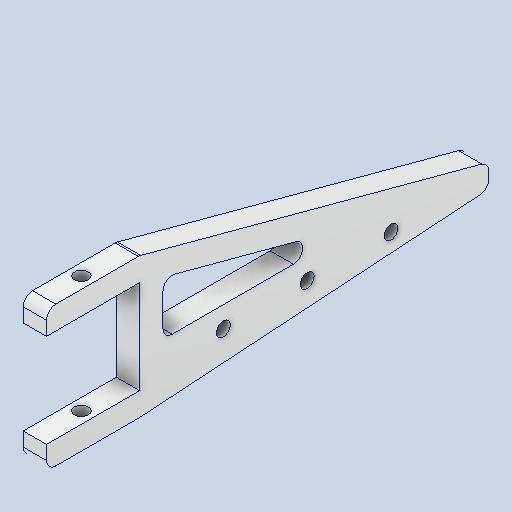
# Autodesk Inventor part: base_weel-v2-Plate-7
Saved by Autodesk Inventor 2025.2 (Build 292293000, 293)
## iProperties
Created: 2025-01-14
Part Number: base_weel-v2-Plate-7
Material: アルミニウム 6061
Document SubType Name: Modeling
Designer: haruy
Density: 2.7 g/cm^3
Appearance: アルミニウム - フラット
Author: haruy
Autodesk Inventor part; units mm, degrees
ref_plane "YZ Plane" through (0, 0, 0) normal (1, 0, 0) x (0, 1, 0)
ref_plane "XZ Plane" through (0, 0, 0) normal (0, 1, 0) x (-1, 0, 0)
ref_plane "XY Plane" through (0, 0, 0) normal (0, 0, 1) x (1, 0, 0)
sketch "スケッチ1" plane through (0, 0, 0) normal (1, 0, 0) x (0, 1, 0)
  line L0 (0, 0) -> (20.1, 0)
  line L1 (20.1, 0) -> (20.1, -20)
  line L2 (20.1, -20) -> (0, -20)
  line L3 (0, -20) -> (0, 0)
  line L4 (0, -20) -> (5, -20)
  line L5 (5, -20) -> (5, -95)
  line L6 (5, -95) -> (0, -95)
  line L7 (0, -95) -> (0, -20)
  circle A0 centre (2.5, -38) radius 1.5
  circle A1 centre (2.5, -56) radius 1.5
  circle A2 centre (2.5, -74) radius 1.5
  line L8 (20.1, 0) -> (25.1, 0)
  line L9 (25.1, 0) -> (25.1, -20)
  line L10 (25.1, -20) -> (20.1, -20)
  line L11 (20.1, -20) -> (20.1, 0)
  line L12 (0, 0) -> (-5, 0)
  line L13 (-5, 0) -> (-5, -20)
  line L14 (-5, -20) -> (0, -20)
  line L15 (0, -20) -> (0, 0)
  line L16 (25.1, -20) -> (5, -95)
  line L17 (-5, -20) -> (0, -95)
  line L18 (25.1, -25) -> (15.1, -25)
  line L19 (15.1, -25) -> (15.1, 0.1)
  line L20 (0, -25) -> (25.1, -25)
  line L21 (25.1, -25) -> (25.1, 0.1)
  line L22 (20.2704, -18.7057) -> (0.1704, -93.7057)
  line L23 (7, -95) -> (7, -18)
  line L24 (7, -18) -> (0, -18)
  line L25 (0, -35) -> (-35, -35)
  line L26 (-35, -35) -> (-35, -85)
  line L27 (-35, -85) -> (0, -85)
  line L28 (0, -85) -> (0, -35)
  line L29 (-35, -38) -> (-70, -38)
  line L30 (-70, -38) -> (-70, -82)
  line L31 (-70, -82) -> (-35, -82)
  line L32 (-35, -82) -> (-35, -38)
  line L33 (7.5, -95) -> (-2.5, -95)
  line L34 (-2.5, -95) -> (-2.5, -21)
  line L35 (-2.5, -21) -> (7.5, -21)
  line L36 (7.5, -21) -> (7.5, -95)
  line L37 (-2.5, -21) -> (-64, -21)
  line L38 (-64, -21) -> (-64, -31)
  line L39 (-64, -31) -> (-2.5, -31)
  line L40 (-2.5, -31) -> (-2.5, -21)
  point P0 (7, -25)
  point P1 (18.5836, -25)
  point P2 (7, -68.2222)
  dimension "d0" = 20.1
  dimension "d1" = 20
  dimension "d2" = 5
  dimension "d3" = 75
  dimension "d4" = 3
  dimension "d5" = 3
  dimension "d6" = 3
  dimension "d7" = 2.5
  dimension "d8" = 2.5
  dimension "d9" = 2.5
  dimension "d10" = 18
  dimension "d11" = 18
  dimension "d12" = 18
  dimension "d13" = 5
  dimension "d14" = 5
  dimension "d15" = 0
  dimension "d16" = 0
  dimension "d17" = 5
  dimension "d18" = 5
  dimension "d19" = 5
  dimension "d20" = 2
  dimension "d33" = 50
  dimension "d34" = 35
  dimension "d35" = 35
  dimension "d36" = 44
  dimension "d37" = 3
  dimension "d38" = 0
  dimension "d39" = 10
  dimension "d40" = 0
  dimension "d41" = 5
  dimension "d42" = 5
  dimension "d43" = 6
  dimension "d44" = 10
  dimension "d46" = 1
  constraints: 82 end point, 17 parallel, 9 perpendicular, 8 horizontal, 3 centre point, 1 point on line, 3 other
  measures "d0" distance of L1.end L2.end
  measures "d1" distance of L0.end L1.end
  measures "d2" distance of L5.end L6.end
  measures "d3" distance between parallel lines of L6 L2
  measures "d4" diameter of A0
  measures "d5" diameter of A1
  measures "d6" diameter of A2
  measures "d7" distance from line of A0.centre L7
  measures "d8" distance from line of A1.centre L7
  measures "d9" distance from line of A2.centre L7
  measures "d10" distance from line of A0.centre L2
  measures "d11" distance of A1.centre A0.centre
  measures "d12" distance of A2.centre A1.centre
  measures "d13" distance of L9.end L10.end
  measures "d14" distance of L14.end L13.end
  measures "d15" distance between parallel lines of L10 L2
  measures "d16" distance between parallel lines of L4 L14
  measures "d17" distance between parallel lines of L10 L18
  measures "d18" distance between parallel lines of L2 L20
  measures "d19" distance between parallel lines of L16 L22
  measures "d20" distance between parallel lines of L5 L23
  measures "d33" distance of L26.end L25.end
  measures "d34" distance of L25.start L25.end
  measures "d35" distance of L31.end L30.end
  measures "d36" distance of L30.end L29.end
  measures "d37" distance between parallel lines of L25 L29
  measures "d38" distance between parallel lines of L7 L28
  measures "d39" distance between parallel lines of L6 L27
  measures "d40" distance between parallel lines of L6 L33
  measures "d41" distance from line of L36 A2.centre
  measures "d42" distance from line of L34 A2.centre
  measures "d43" distance between parallel lines of L30 L38
  measures "d44" distance between parallel lines of L39 L37
  measures "d46" distance between parallel lines of L35 L4
extrude "押し出し1" add sketch "スケッチ1" against normal blind 5 contours L3 L14 L13 L12 | L8 L9 L10 L1 | L19 L20 L36 L35 L23 L2 | L2 L22 L18 L19 | L2 L5 L35 L7 | L7 L35 L37 L17 L14 | L2 L10 L16 L18 L22 | L23 L35 L5 L2 | L35 L5 L20 L7 | L7 L25 L34 L35 | L37 L34 L39 L17 | L18 L16 L36 L22 | L35 L36 L20 L23 | L23 L20 L5 L35 | L20 L5 L6 L7 | L39 L34 L25 L17 | L36 L16 L23 L22 | L23 L22 L5 L20 | L7 L27 L17 L34 L25 | L25 L34 L17 | L23 L16 L5 L22 | L7 L17 L27
fillet "フィレット1" radius 2 9 edges at (-2.5, 7, -25) (-2.5, 18.5836, -25) (-2.5, 7, -68.2222) (-2.5, 25.1, 0) (-2.5, 25.1, -20) (-2.5, -5, 0) (-2.5, -5, -20) (-2.5, 0, -95) (-2.5, 5, -95)
sketch "スケッチ2" plane through (0, 25.1, 0) normal (0, 1, 0) x (1, 0, 0)
  line L0 (0, 0) -> (-5, 0) projected
  line L1 (-5, 2) -> (-5, 19.7366) projected
  point P0 (-2.5, 10)
  point P1 (-5, 20.1)
  dimension "d24" = 10
  dimension "d25" = 2.5
  measures "d24" distance from line of L0 point (-2.5, 10)
  measures "d25" distance from line of point (-2.5, 10) L1
hole "穴1" at (-2.5, 25.1, -10) direction (0, -1, 0) diameter 3 end through all
equation "\"d8\" = d7"
equation "\"d9\" = d7"
equation "\"d11\" = d10"
equation "\"d12\" = d10"
